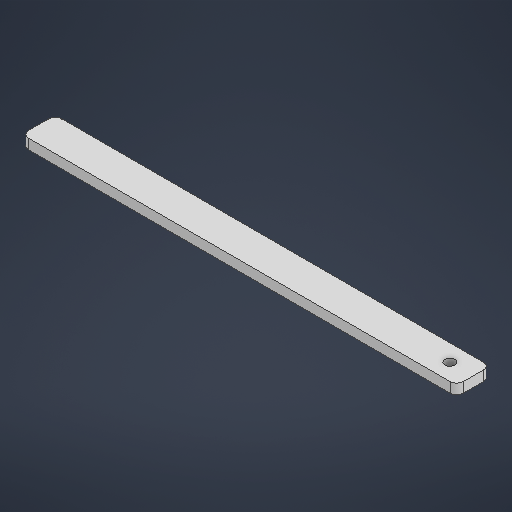
# Autodesk Inventor part: Brazo_Servo
Saved by Autodesk Inventor 2026 (Build 300175000, 175)
## iProperties
Created: 2025-06-18
Part Number: Brazo_Servo
Material: Genérico
Document SubType Name: Modeling
Designer: oscar
Density: 1 g/cm^3
Appearance: Valor por defecto
Author: oscar
Autodesk Inventor part; units mm, degrees
ref_plane "YZ Plane" through (0, 0, 0) normal (1, 0, 0) x (0, 1, 0)
ref_plane "XZ Plane" through (0, 0, 0) normal (0, 1, 0) x (-1, 0, 0)
ref_plane "XY Plane" through (0, 0, 0) normal (0, 0, 1) x (1, 0, 0)
sketch "Boceto1" plane through (0, 0, 0) normal (0, 1, 0) x (-1, 0, 0)
  line L0 (65, 5) -> (-65, 5)
  line L1 (-65, 5) -> (-65, -5)
  line L2 (-65, -5) -> (65, -5)
  line L3 (65, -5) -> (65, 5)
  line L4 (65, 5) -> (-65, -5) construction
  line L5 (-65, 5) -> (65, -5) construction
  point P0 (0, 0)
  dimension "d0" = 130
  dimension "d1" = 10
  constraints: 12 end point, 2 midpoint, 2 parallel, 1 horizontal, 1 perpendicular
  measures "d0" distance of L2.end L1.end
  measures "d1" distance of L1.end L0.end
extrude "Extrusión1" add sketch "Boceto1" along normal blind 3
sketch "Boceto2" plane through (0, 3, 0) normal (0, 1, 0) x (1, 0, 0)
  circle A0 centre (58, 0) radius 1.5
  line L0 (65, 5) -> (-65, 5) projected
  line L1 (65, -5) -> (65, 5) projected
  point P0 (0, 0)
  point P1 (65, 0)
  point P2 (65, 0)
  dimension "d4" = 3
  dimension "d5" = 5
  dimension "d7" = 7
  constraints: 2 midpoint, 1 centre point
  measures "d4" diameter of A0
  measures "d5" distance from line of L0 A0.centre
  measures "d7" distance of point (65, 0) A0.centre
extrude "Extrusión2" cut sketch "Boceto2" against normal blind 3
fillet "Empalme1" radius 2 1 edges at (-65, 1.5, 5)
fillet "Empalme2" radius 2 1 edges at (-65, 1.5, -5)
fillet "Empalme3" radius 2 1 edges at (65, 1.5, 5)
fillet "Empalme4" radius 2 1 edges at (65, 1.5, -5)
